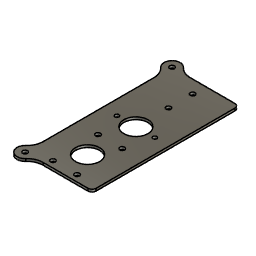
4_Fuerza v3 (Autodesk Fusion 360 design; units mm, degrees)
Autodesk Fusion 360 part; units mm, degrees
note: some values were not read from the file. Set by a fixed rule: which sketch regions a step uses.
sketch "Sketch1" plane through (0, 0, 0) normal (0, 0, 1) x (1, 0, 0)
  line L0 (99.5, 80) -> (40.5, 80)
  line L1 (40.5, 80) -> (40.5, 10)
  line L2 (40.5, 10) -> (99.5, 10)
  line L3 (99.5, 10) -> (99.5, 80)
  line L4 (99.5, 80) -> (40.5, 10) construction
  line L5 (40.5, 80) -> (99.5, 10) construction
  line L6 (40.5, 73) -> (100, 73) construction
  line L7 (70, 45) -> (70, 80) construction
  circle A0 centre (55, 73) radius 3
  circle A1 centre (85, 73) radius 3
  line L8 (70, 45) -> (40, 45) construction
  circle A2 centre (55, 17) radius 3
  circle A3 centre (85, 17) radius 3
  circle A4 centre (70, 45) radius 15
  line L9 (101.5, 127.5) -> (38.5, 82.5) construction
  line L10 (101.5, 82.5) -> (38.5, 127.5) construction
  line L11 (101.5, 127.5) -> (38.5, 127.5)
  line L12 (101.5, 82.5) -> (101.5, 127.5)
  line L13 (38.5, 82.5) -> (101.5, 82.5)
  line L14 (38.5, 127.5) -> (38.5, 82.5)
  circle A5 centre (46.5, 105) radius 2.5
  circle A6 centre (70, 105) radius 15
  circle A7 centre (93.5, 105) radius 2.5
  line L15 (70, 80) -> (70, 120) construction
  line L16 (45.0759, 190.4025) -> (95.0759, 190.4025)
  line L17 (95.0759, 190.4025) -> (95.0759, 130.4025)
  line L18 (95.0759, 130.4025) -> (45.0759, 130.4025)
  line L19 (45.0759, 130.4025) -> (45.0759, 190.4025)
  line L20 (70.0759, 190.4025) -> (70.0759, 130.4025) construction
  line L21 (70.0759, 160.4025) -> (95.0759, 160.4025) construction
  circle A8 centre (70.0759, 175.4025) radius 3
  circle A9 centre (70.0759, 145.4025) radius 3
  line L22 (28.5, 191.4025) -> (28.5, 9)
  line L23 (111.5, 191.4025) -> (111.5, 9)
  line L24 (28.5, 191.4025) -> (111.5, 191.4025)
  line L25 (28.5, 9) -> (111.5, 9)
  circle A10 centre (28.5, 191.4025) radius 3
  circle A11 centre (28.5, 191.4025) radius 10
  circle A12 centre (28.5, 9) radius 3
  circle A13 centre (28.5, 9) radius 10
  point P0 (70, 45)
  dimension "d1" = 59
  dimension "d2" = 70
  dimension "d3" = 7
  dimension "d5" = 6
  dimension "d6" = 15
  dimension "d7" = 30
  dimension "d8" = 45
  dimension "d9" = 63
  dimension "d10" = 5
  dimension "d11" = 30
  dimension "d12" = 50
  dimension "d13" = 60
  dimension "d14" = 6
  dimension "d15" = 15
  dimension "d16" = 10
  dimension "d17" = 10
  dimension "d18" = 1
  dimension "d19" = 1
  dimension "d22" = 6
  dimension "d23" = 20
  dimension "d24" = 6
  dimension "d25" = 20
  constraint horizontal L0
  constraint perpendicular L0 L1
  constraint parallel L0 L2
  constraint parallel L1 L3
  constraint coincident L4 P0
  constraint coincident L5 P0
  constraint coincident L1 L6.start
  constraint perpendicular L1 L6
  constraint coincident P0 L7.start
  constraint midpoint L0 L7.end
  constraint coincident L6 A0.centre
  constraint symmetric L7 A0 A1
  constraint perpendicular L7 L8
  constraint symmetric A0 L8 A2
  constraint symmetric A1 L8 A3
  constraint perpendicular L11 L12
  constraint parallel L12 L14
  constraint parallel L11 L13
  constraint perpendicular L0 L15
  constraint horizontal L16
  constraint vertical L17
  constraint horizontal L18
  constraint vertical L19
  constraint midpoint L16 L20.start
  constraint midpoint L18 L20.end
  constraint midpoint L20 L21.start
  constraint midpoint L17 L21.end
  constraint coincident L20 A8.centre
  constraint symmetric L21 A8 A9
  constraint vertical L22
  constraint vertical L23
  constraint perpendicular L23 L24
  constraint perpendicular L23 L25
  constraint coincident L22.start L24.start
  constraint concentric A10 A11
  constraint coincident L22.end L25.start
  constraint concentric A12 A13
  measures "d1" distance of L1.end L2.end
  measures "d2" distance of L0.end L1.end
  measures "d3" distance of L0 L6
  measures "d5" diameter of A0
  measures "d6" distance of L7 A0.centre
  measures "d7" diameter of A4
  measures "d8" distance of L10.end L9.end
  measures "d9" distance of L10.end L9.start
  measures "d10" diameter of A7
  measures "d11" diameter of A6
  measures "d12" distance of L16.start L16.end
  measures "d13" distance of L16.start L18.end
  measures "d14" diameter of A8
  measures "d15" distance of L21 A8.centre
  measures "d16" distance of L14 L22
  measures "d17" distance of L12 L23
  measures "d18" distance of L16 L24
  measures "d19" distance of L2 L25
  measures "d22" diameter of A10
  measures "d23" diameter of A11
  measures "d24" diameter of A12
  measures "d25" diameter of A13
extrude "Extrude1" add sketch "Sketch1" along normal blind 3 contours L0 L1 L2 L3 | L11 L12 L13 L14 | L16 L17 L18 L19 | L22 L24 A10 A11 | L22 L24 A10 A11 | L22 L23 L24 L25 A11 A13 | L22 L25 A12 A13 | L22 L25 A12 A13
fillet "Fillet1" radius 20 2 edges at (38.5, 191.4025, 1.5) (28.5, 181.4025, 1.5)
fillet "Fillet2" radius 20 2 edges at (38.5, 9, 1.5) (28.5, 19, 1.5)
fillet "Fillet3" radius 5 2 edges at (111.5, 191.4025, 1.5) (111.5, 9, 1.5)
equation "d17 = d16"
